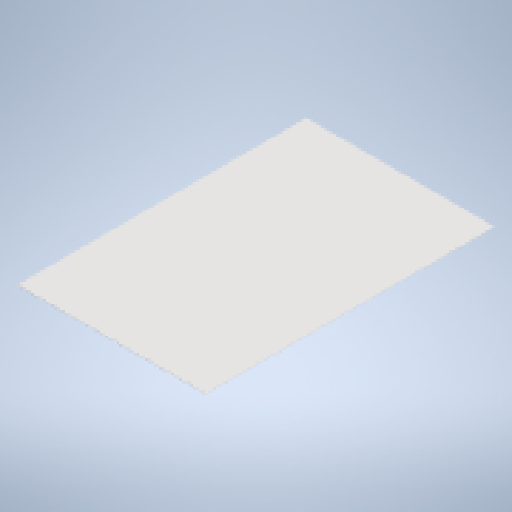
# Autodesk Inventor part: BSH 010 floor 1
Saved by Autodesk Inventor 2025 (Build 290162010, 162A)
## iProperties
Created: 2024-07-23
Part Number: BSH 010 floor 1
Material: Steel
Document SubType Name: Sheet Metal
Designer: admin
Density: 7.85 g/cm^3
Sheet Metal Rule: AISI304 3mm Die 32
Appearance: Default
Author: admin
Autodesk Inventor part; units mm, degrees
ref_plane "YZ Plane" through (0, 0, 0) normal (1, 0, 0) x (0, 1, 0)
ref_plane "XZ Plane" through (0, 0, 0) normal (0, 1, 0) x (-1, 0, 0)
ref_plane "XY Plane" through (0, 0, 0) normal (0, 0, 1) x (1, 0, 0)
sketch "Sketch1" plane through (0, 0, 0) normal (0, 0, 1) x (1, 0, 0)
  line L0 (-625, -950) -> (625, -950)
  line L1 (625, -950) -> (625, 950)
  line L2 (625, 950) -> (-625, 950)
  line L3 (-625, 950) -> (-625, -950)
  line L4 (-625, -950) -> (625, 950) construction
  line L5 (625, -950) -> (-625, 950) construction
  point P0 (0, 0)
  dimension "d0" = 1250
  dimension "d1" = 1900
  measures "d0" distance of L2.end L1.end
  measures "d1" distance of L1.end L0.end
extrude "Plate1" add sketch "Sketch1" along normal blind 3
sketch "Sketch2" plane through (625, 947.8787, 0.8787) normal (0, 0.7071068, 0.7071068) x (-1, 0, 0)
  line L0 (1250, 0) -> (0, 0)
  line L1 (0, 0) -> (0, -212)
  line L2 (0, -212) -> (1250, -212)
  line L3 (1250, -212) -> (1250, 0)
  constraints: 6 end point, 1 horizontal, 1 perpendicular, 1 vertical
edge flange "Flange1" height 212 angle 45 thickness 3 bend radius 5 thickness toward (0, 0.7071068, 0.7071068) relief round relief width 3 relief depth 1.5 corner gap 5 corner form 0 edges at (0, 950, 0) (0, -950, 0) wall of the first edge with corners at (-625, 947.8787, 0.8787) (625, 947.8787, 0.8787) (625, 1097.7853, -149.028) (-625, 1097.7853, -149.028)
bend "Bend1"
corner "Corner1"
equation "\"d2\" = Thickness"
equation "\"d3\" = BendReliefWidth"
equation "\"d4\" = BendReliefDepth"
equation "\"d5\" = MinimumRemnant"
equation "\"d6\" = TransitionRadius"
equation "\"d9\" = BendRadius"
equation "\"d10\" = CornerReliefSize"
equation "\"d11\" = GapSize"
equation "\"d12\" = JacobiRadiusSize"
equation "\"BendReliefWidth\" = Thickness"
equation "\"BendReliefDepth\" = 0.5 * Thickness"
equation "\"CornerReliefSize\" = 4 * Thickness"
equation "\"MinimumRemnant\" = 2 * Thickness"
equation "\"TransitionRadius\" = BendRadius"
equation "\"JacobiRadiusSize\" = BendRadius"
equation "\"GapSize\" = Thickness"
equation "\"Thickness\" = 3"
equation "\"BendRadius\" = 5"
body "Solid1"
